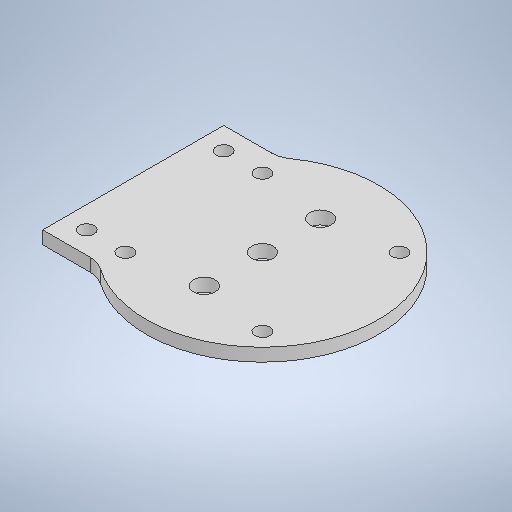
# Autodesk Inventor part: SCARA arm base - lid
Saved by Autodesk Inventor 2025.2 (Build 292293000, 293)
## iProperties
Created: 2025-01-29
Part Number: SCARA arm base - lid
Material: Generic
Document SubType Name: Modeling
Designer: caomi
Density: 1 g/cm^3
Appearance: Default
Author: caomi
Autodesk Inventor part; units mm, degrees
ref_plane "YZ Plane" through (0, 0, 0) normal (1, 0, 0) x (0, 1, 0)
ref_plane "XZ Plane" through (0, 0, 0) normal (0, 1, 0) x (-1, 0, 0)
ref_plane "XY Plane" through (0, 0, 0) normal (0, 0, 1) x (1, 0, 0)
sketch "Sketch1" plane through (0, 0, 0) normal (0, 1, 0) x (-1, 0, 0)
  circle A0 centre (0, 0) radius 45
  line L0 (28.2843, 35) -> (50, 35)
  line L1 (50, 35) -> (50, -35)
  line L2 (50, -35) -> (28.2843, -35)
  dimension "d0" = 90
  dimension "d1" = 70
  dimension "d2" = 50
  constraints: 6 end point, 2 perpendicular, 2 point on circle, 1 centre point, 1 coincident, 1 horizontal, 1 vertical alignment
  measures "d0" diameter of A0
  measures "d1" distance of L0.end L1.end
  measures "d2" distance from line of point (0, 0) L1
extrude "Extrusion1" add sketch "Sketch1" along normal blind 5
fillet "Fillet1" radius 10 2 edges at (-28.2843, 2.5, 35) (-28.2843, 2.5, -35)
sketch "Sketch2" plane through (0, 5, 0) normal (0, 1, 0) x (1, 0, 0)
  line L0 (0, 0) -> (-26.5165, -26.5165) construction
  line L1 (0, 0) -> (0, -28.6584) construction
  line L2 (0, 0) -> (-21.9625, 0) construction
  point P0 (-41.5165, -26.5165)
  point P1 (26.5165, -26.5165)
  point P2 (-26.5165, 26.5165)
  point P3 (-41.5165, 26.5165)
  point P4 (26.5165, 26.5165)
  dimension "d6" = 45
  dimension "d7" = 37.5
  dimension "d8" = 15
  constraints: 6 end point, 4 symmetric about line, 1 coincident, 1 horizontal, 1 horizontal alignment, 1 vertical
  measures "d6" angle of L1 L0
  measures "d7" distance of L0.start L0.end
  measures "d8" distance of L0.end point (-41.517, -26.517)
hole "Hole1" at (-26.5165, 5, 26.5165) at (-41.5165, 5, 26.5165) at (-41.5165, 5, -26.5165) at (26.5165, 5, 26.5165) at (26.5165, 5, -26.5165) at (-26.5165, 5, -26.5165) direction (0, -1, 0) diameter 4.3 end through all counterbore diameter 5.8 counterbore depth 4
sketch "Sketch3" plane through (0, 5, 0) normal (0, 1, 0) x (1, 0, 0)
  circle A0 centre (0, 0) radius 4.15
  circle A1 centre (0, -22.5) radius 4.15
  circle A2 centre (0, 22.5) radius 4.15
  line L0 (-69, 0) -> (64, 0) projected
  dimension "d16" = 45
  dimension "d17" = 8.3
  constraints: 3 centre point, 2 equal radius, 1 coincident, 1 symmetric about line, 1 vertical alignment
  measures "d16" distance of A2.centre A1.centre
  measures "d17" diameter of A0
extrude "Extrusion2" cut sketch "Sketch3" against normal blind 8.3
equation "\"d18\" = d17"
body "Solid1"
